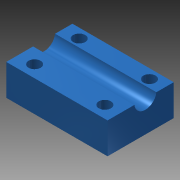
# Autodesk Inventor part: YMotorCapLeft
Saved by Autodesk Inventor 2015 SP1 (Build 190203100, 203)
## iProperties
Created: 2014-08-15
Part Number: YMotorCapLeft
Material: ABS Plastic
Document SubType Name: Modeling
Designer: t_clevj
Density: 1.06 g/cm^3
Appearance: Cyan
Mass: 9.67654 g
Surface Area: 40.7284 cm^2
Volume: 9.12882 cm^3
Author: Jack; Zelogik
Autodesk Inventor part; units mm, degrees
ref_plane "YZ Plane" through (0, 0, 0) normal (1, 0, 0) x (0, 1, 0)
ref_plane "XZ Plane" through (0, 0, 0) normal (0, 1, 0) x (-1, 0, 0)
ref_plane "XY Plane" through (0, 0, 0) normal (0, 0, 1) x (1, 0, 0)
sketch "Sketch1" plane through (0, 0, 0) normal (0, 0, 1) x (1, 0, 0)
  line L0 (0, 0) -> (37.5, 0)
  line L1 (37.5, 0) -> (37.5, 24.5)
  line L2 (37.5, 24.5) -> (0, 24.5)
  line L3 (0, 24.5) -> (0, 0)
  dimension "d0" = 37.5
  dimension "d1" = 24.5
  constraints: 8 end point, 2 parallel, 1 horizontal, 1 perpendicular
  measures "d0" distance of L2.end L1.end
  measures "d1" distance of L1.end L0.end
extrude "Extrusion1" add sketch "Sketch1" along normal blind 11.5
sketch "Sketch2" plane through (0, 0, 0) normal (-1, 0, 0) x (0, 0, 1)
  line L0 (11.5, 24.5) -> (11.5, 0) projected
  line L1 (0, 24.5) -> (11.5, 24.5) projected
  circle A0 centre (12, 14.5) radius 4.1
  dimension "d4" = 8.2
  dimension "d5" = 0.5
  dimension "d6" = 10
  constraints: 1 centre point
  measures "d4" diameter of A0
  measures "d5" distance from line of L0 A0.centre
  measures "d6" distance from line of L1 A0.centre
extrude "Extrusion2" cut sketch "Sketch2" against normal up to surface (37.5 mm away)
sketch "Sketch3" plane through (0, 0, 0) normal (0, 0, -1) x (-1, 0, 0)
  line L0 (0, 24.5) -> (0, 0) projected
  line L1 (0, 18.5694) -> (0, 10.4306) projected
  line L2 (0, 0) -> (-37.5, 0) projected
  point P0 (-6, 21)
  point P1 (-32, 21)
  point P2 (-32, 4.5)
  point P3 (-6, 4.5)
  dimension "d9" = 6
  dimension "d10" = 32
  dimension "d30" = 4.5
  dimension "d32" = 21
  constraints: 2 horizontal alignment, 2 vertical alignment
  measures "d9" distance from line of L0 point (-6, 21)
  measures "d10" distance from line of point (-32, 21) L0
  measures "d30" distance from line of L2 point (-6, 4.5)
  measures "d32" distance from line of L2 point (-6, 21)
hole "Hole1" at (6, 21, 0) at (32, 21, 0) at (32, 4.5, 0) at (6, 4.5, 0) direction (0, 0, 1) diameter 4.5 depth 11.5 tip angle 118 counterbore diameter 8 counterbore depth 4
body "Solid1"
